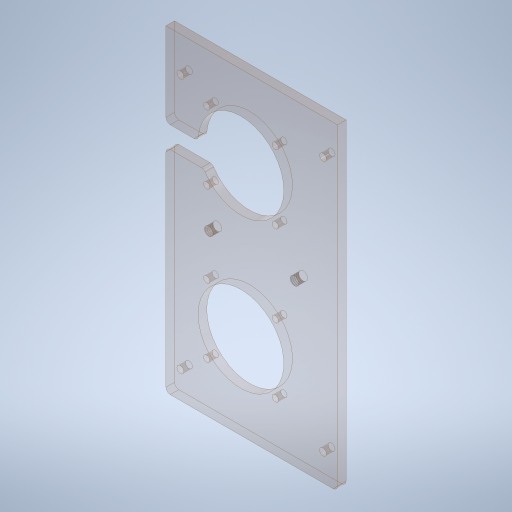
# Autodesk Inventor part: Placa soporte TIC DC
Saved by Autodesk Inventor 2024.2 (Build 282272000, 272)
## iProperties
Created: 2024-08-28
Part Number: Placa soporte TIC DC
Material: Polycarbonate, Smoke
Document SubType Name: Modeling
Designer: ja.restrepo1
Density: 1.2 g/cm^3
Appearance: Polycarbonate - Smoked
Author: ja.restrepo1
Autodesk Inventor part; units mm, degrees
ref_plane "YZ Plane" through (0, 0, 0) normal (1, 0, 0) x (0, 1, 0)
ref_plane "XZ Plane" through (0, 0, 0) normal (0, 1, 0) x (-1, 0, 0)
ref_plane "XY Plane" through (0, 0, 0) normal (0, 0, 1) x (1, 0, 0)
sketch "Sketch1" plane through (0, 0, 0) normal (0, 0, 1) x (-1, 0, 0)
  line L0 (-38, 74) -> (38, 74)
  line L1 (40, 72) -> (40, -74)
  line L2 (40, -74) -> (-40, -74)
  line L3 (-40, -74) -> (-40, 72)
  circle A0 centre (-33.25, 61.5) radius 1.65
  circle A1 centre (33.25, 61.5) radius 1.65
  circle A2 centre (33.25, -57.5) radius 1.65
  circle A3 centre (-33.25, -57.5) radius 1.65
  line L4 (-33.25, 61.5) -> (33.25, 61.5) construction
  line L5 (33.25, 61.5) -> (33.25, -57.5) construction
  circle A4 centre (5, 35) radius 20
  circle A5 centre (5, -35) radius 20
  line L6 (5, 35) -> (5, -35) construction
  line L7 (-11, -51) -> (21, -51) construction
  line L8 (21, -51) -> (21, -19) construction
  line L9 (-11, 51) -> (21, 51) construction
  line L10 (21, 51) -> (21, 19) construction
  circle A6 centre (-11, 51) radius 1.5
  circle A7 centre (21, 51) radius 1.5
  circle A8 centre (21, 19) radius 1.5
  circle A9 centre (-11, 19) radius 1.5
  circle A10 centre (21, -19) radius 1.5
  circle A11 centre (21, -51) radius 1.5
  circle A12 centre (-11, -51) radius 1.5
  circle A13 centre (-11, -19) radius 1.5
  arc A14 (-38, 74) -> (-40, 72) centre (-38, 72) ccw
  arc A15 (40, 72) -> (38, 74) centre (38, 72) ccw
  point P0 (0, 0)
  point P1 (-40, 74)
  point P2 (40, 74)
  point P3 (0, 74)
  point P4 (-40, 0)
  point P5 (0, 61.5)
  point P6 (5, 0)
  point P7 (21, 35)
  point P8 (5, 51)
  point P9 (5, -51)
  point P10 (21, -35)
  dimension "d15" = 2
  dimension "d0" = 80
  dimension "d1" = 148
  dimension "d2" = 3.3
  dimension "d3" = 119
  dimension "d4" = 66.5
  dimension "d20" = 40
  dimension "d21" = 40
  dimension "d22" = 70
  dimension "d23" = 32
  dimension "d24" = 3
  dimension "d26" = 5
  dimension "d28" = 2
  dimension "d29" = 16.5
  dimension "d30" = 74
  constraints: 22 end point, 16 centre point, 11 equal radius, 11 vertical alignment, 9 horizontal alignment, 7 midpoint, 6 coincident, 5 point on line, 4 point on circle, 4 tangent, 3 horizontal, 2 equal length, 2 parallel, 2 perpendicular, 2 vertical
  measures "d0" distance of L2.end L1.end
  measures "d1" distance of L1.end point (40, 74)
  measures "d2" diameter of A0
  measures "d3" distance of L4.end L5.end
  measures "d4" distance of L4.start L4.end
  measures "d20" diameter of A4
  measures "d21" diameter of A5
  measures "d22" distance of L6.start L6.end
  measures "d23" distance of L7.start L7.end
  measures "d24" diameter of A6
  measures "d26" distance from line of L6 point (0, 0)
  measures "d28" radius of A14
  measures "d29" distance from line of A3.centre L2
  measures "d30" distance from line of point (0, 0) L2
extrude "soporte circuito KAEN" add sketch "Sketch1" along normal mid plane 4
sketch "Sketch2" plane through (0, 0, 2) normal (0, 0, 1) x (-1, 0, 0)
  line L0 (-20, -1) -> (20, -1) construction
  line L1 (40, -74) -> (40, 72) construction
  line L2 (-40, -74) -> (40, -74) projected
  point P0 (0, 0)
  point P1 (36.5, 73)
  point P2 (0, -1)
  point P3 (36.5, -74)
  point P4 (-36.5, -74)
  point P5 (34.5, -75)
  point P6 (40, 72)
  dimension "d11" = 40
  dimension "d25" = 73
  constraints: 2 end point, 1 horizontal, 1 midpoint, 1 vertical alignment, 2 other
  measures "d11" distance of L0.start L0.end
hole "M5" at (20, 1, 2) at (-20, 1, 2) direction (0, 0, -1) diameter 4.134 end through all thread size "M5x0.8" class "6H" standard "ANSI Metric M Profile"
sketch "Sketch3" plane through (0, 0, 2) normal (0, 0, 1) x (1, 0, 0)
  line L0 (-41, 35) -> (-22, 35)
  line L1 (-22, 35) -> (-22, 25)
  line L2 (-22, 25) -> (-41, 25)
  line L3 (-41, 25) -> (-41, 35)
  circle A0 centre (-5, 35) radius 20 projected
  point P0 (0, 0)
  point P1 (-31.5, 35)
  point P2 (-22.3205, 25)
  point P3 (-25, 35)
  dimension "d31" = 10
  dimension "d32" = 19
  dimension "d33" = 17
  constraints: 8 end point, 2 parallel, 1 horizontal, 1 horizontal alignment, 1 midpoint, 1 perpendicular
  measures "d31" distance of L2.end L0.start
  measures "d32" distance of L1.end L2.end
  measures "d33" distance from line of A0.centre L1
extrude "Extrusion2" cut sketch "Sketch3" against normal through all contours L0 A0 L2 L3
fillet "Fillet2" radius 2 4 edges at (-40, 35, 0) (-40, 25, 0) (-25, 35, 0) (-22.3205, 25, 0)
body "Solid1"
